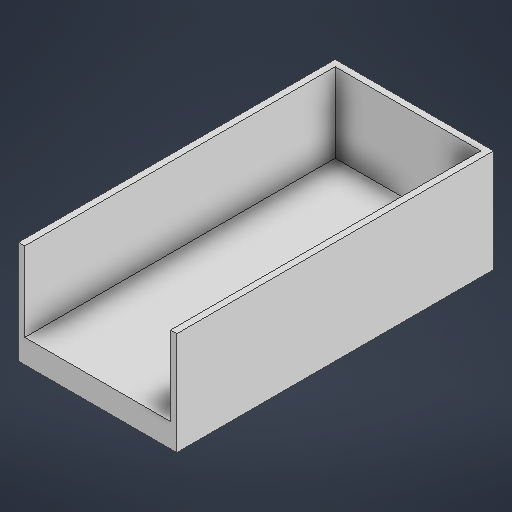
# Autodesk Inventor part: electronics tray
Saved by Autodesk Inventor 2026.1 (Build 301233000, 233)
## iProperties
Created: 2025-11-07
Part Number: electronics tray
Material: Generic
Document SubType Name: Modeling
Designer: Ethan
Density: 1 g/cm^3
Appearance: Default
Author: Ethan
Autodesk Inventor part; units mm, degrees
ref_plane "YZ Plane" through (0, 0, 0) normal (1, 0, 0) x (0, 1, 0)
ref_plane "XZ Plane" through (0, 0, 0) normal (0, 1, 0) x (-1, 0, 0)
ref_plane "XY Plane" through (0, 0, 0) normal (0, 0, 1) x (1, 0, 0)
sketch "Sketch1" plane through (0, 0, 0) normal (0, 1, 0) x (-1, 0, 0)
  line L0 (0, 0) -> (100, 0)
  line L1 (100, 0) -> (100, 200)
  line L2 (100, 200) -> (0, 200)
  line L3 (0, 200) -> (0, 0)
  dimension "d0" = 200
  dimension "d1" = 100
  constraints: 8 end point, 2 parallel, 1 horizontal, 1 perpendicular
  measures "d0" distance of L0.end L1.end
  measures "d1" distance of L1.end L2.end
extrude "Extrusion1" add sketch "Sketch1" along normal blind 5
sketch "Sketch2" plane through (0, 5, 0) normal (0, 1, 0) x (1, 0, 0)
  line L0 (-100, -200) -> (0, -200) projected
  line L1 (0, -200) -> (0, 0) projected
  line L2 (-100, -200) -> (0, -200)
  line L3 (0, -200) -> (0, 0)
  line L4 (0, 0) -> (-100, 0)
  line L5 (-100, 0) -> (-100, -200)
  line L6 (-96, -196) -> (-4, -196)
  line L7 (-4, -196) -> (-4, -4)
  line L8 (-4, -4) -> (-96, -4)
  line L9 (-96, -4) -> (-96, -196)
  dimension "d4" = 4
  constraints: 16 end point, 4 parallel, 2 perpendicular, 1 horizontal, 3 other
  measures "d4" distance between parallel lines of L5 L9
extrude "Extrusion2" add sketch "Sketch2" along normal blind 50
sketch "Sketch3" plane through (-100, 0, 200) normal (0, 0, 1) x (1, 0, 0)
  line L0 (96, 5) -> (96, 55) projected
  line L1 (96, 5) -> (4, 5) projected
  line L2 (96, 55) -> (4, 55)
  line L3 (4, 55) -> (4, 5)
  line L4 (4, 5) -> (96, 5)
  line L5 (96, 5) -> (96, 55)
  point P0 (100, 0)
  constraints: 8 end point, 2 parallel, 1 horizontal, 1 perpendicular
extrude "Extrusion3" cut sketch "Sketch3" against normal blind 50
sketch "Sketch4" plane through (0, 0, 0) normal (0, -1, 0) x (1, 0, 0)
  line L0 (-100, 0) -> (-100, 200) projected
  line L1 (-100, 200) -> (0, 200)
  line L2 (0, 200) -> (0, 0)
  line L3 (0, 0) -> (-100, 0)
  line L4 (-100, 0) -> (-100, 200)
  line L5 (-4, 4) -> (-4, 200) projected
  line L6 (-96, 200) -> (-96, 4) projected
  line L7 (-4, 4) -> (-96, 4)
  line L8 (-96, 4) -> (-96, 195)
  line L9 (-96, 195) -> (-4, 195)
  line L10 (-4, 195) -> (-4, 4)
  point P0 (-4, 195)
  dimension "d9" = 5
  constraints: 16 end point, 4 parallel, 2 horizontal, 2 perpendicular, 1 point on line
  measures "d9" distance between parallel lines of L1 L9
extrude "Extrusion4" add sketch "Sketch4" along normal blind 10 contours L0 L1 L6 L7 L5 L2 L3 | L1 L5 L9 L6
body "Solid1"
